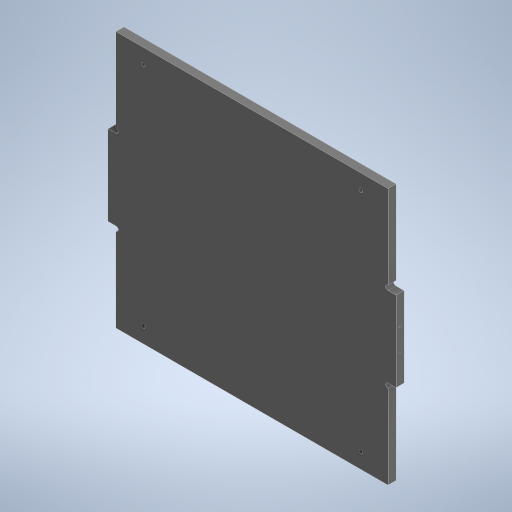
# Autodesk Inventor part: TorsoCoverFrameBasis
Saved by Autodesk Inventor 2024.2 (Build 282272000, 272)
## iProperties
Created: 2024-01-05
Part Number: TorsoCoverFrameBasis
Material: Acetal Resin, Black
Document SubType Name: Modeling
Designer: Masato Kubotera
Density: 1.425 g/cm^3
Appearance: Gray
Vendor: meviy
Mass: 132.259 g
Surface Area: 403.156 cm^2
Volume: 92.813 cm^3
Author: Masato Kubotera
Autodesk Inventor part; units mm, degrees
ref_plane "YZ Plane" through (0, 0, 0) normal (1, 0, 0) x (0, 1, 0)
ref_plane "XZ Plane" through (0, 0, 0) normal (0, 1, 0) x (-1, 0, 0)
ref_plane "XY Plane" through (0, 0, 0) normal (0, 0, 1) x (1, 0, 0)
sketch "Sketch1" plane through (0, 0, 0) normal (1, 0, 0) x (0, 1, 0)
  line L0 (-90, 80.25) -> (90, 80.25)
  line L1 (90, 80.25) -> (90, -80.25)
  line L2 (90, -80.25) -> (-90, -80.25)
  line L3 (-90, -80.25) -> (-90, 80.25)
  line L4 (-90, 80.25) -> (90, -80.25) construction
  line L5 (90, 80.25) -> (-90, -80.25) construction
  line L6 (85, 80.25) -> (85, 25)
  line L7 (85, 25) -> (90, 25)
  line L8 (0, 80.25) -> (0, -80.25)
  line L9 (90, 0) -> (-90, 0) construction
  arc A0 (85, 28) -> (85, 25) centre (85, 26.5) ccw
  line L10 (85, -80.25) -> (85, -25)
  line L11 (85, -25) -> (90, -25)
  arc A1 (85, -25) -> (85, -28) centre (85, -26.5) ccw
  line L12 (-90, 80.25) -> (-90, -80.25)
  line L13 (-85, 80.25) -> (-85, 25)
  line L14 (-85, 25) -> (-90, 25)
  arc A2 (-85, 25) -> (-85, 28) centre (-85, 26.5) ccw
  line L15 (-85, -80.25) -> (-85, -25)
  line L16 (-85, -25) -> (-90, -25)
  arc A3 (-85, -28) -> (-85, -25) centre (-85, -26.5) ccw
  circle A4 centre (68, 70.75) radius 3 construction
  arc A5 (68, 72.85) -> (68, 68.65) centre (68, 70.75) ccw construction
  line L17 (68, 72.85) -> (71.5201, 72.85) construction
  arc A6 (71.5201, 68.65) -> (71.5201, 72.85) centre (75.5, 70.75) ccw construction
  line L18 (68, 70.75) -> (75.5, 70.75) construction
  line L19 (68, 68.65) -> (71.5201, 68.65) construction
  circle A7 centre (68, -70.75) radius 3 construction
  arc A8 (68, -68.65) -> (68, -72.85) centre (68, -70.75) ccw construction
  line L20 (68, -72.85) -> (71.5201, -72.85) construction
  arc A9 (71.5201, -72.85) -> (71.5201, -68.65) centre (75.5, -70.75) ccw construction
  line L21 (68, -70.75) -> (75.5, -70.75) construction
  line L22 (68, -68.65) -> (71.5201, -68.65) construction
  circle A10 centre (-68, 70.75) radius 3 construction
  arc A11 (-68, 68.65) -> (-68, 72.85) centre (-68, 70.75) ccw construction
  line L23 (-68, 72.85) -> (-71.5201, 72.85) construction
  arc A12 (-71.5201, 72.85) -> (-71.5201, 68.65) centre (-75.5, 70.75) ccw construction
  line L24 (-68, 70.75) -> (-75.5, 70.75) construction
  line L25 (-68, 68.65) -> (-71.5201, 68.65) construction
  arc A13 (-68, -72.85) -> (-68, -68.65) centre (-68, -70.75) ccw construction
  circle A14 centre (-68, -70.75) radius 3 construction
  line L26 (-68, -72.85) -> (-71.5201, -72.85) construction
  line L27 (-68, -70.75) -> (-75.5, -70.75) construction
  arc A15 (-71.5201, -68.65) -> (-71.5201, -72.85) centre (-75.5, -70.75) ccw construction
  line L28 (-68, -68.65) -> (-71.5201, -68.65) construction
  line L29 (90, 7) -> (85, 7) construction
  line L30 (90, -7) -> (85, -7) construction
  line L31 (28.3579, -70.25) -> (-28.3579, -70.25)
  line L32 (31.8934, -71.7145) -> (40.4289, -80.25)
  line L33 (-31.8934, -71.7145) -> (-40.4289, -80.25)
  arc A16 (38.9645, -78.7855) -> (42.5, -80.25) centre (42.5, -75.25) ccw
  arc A17 (31.8934, -71.7145) -> (28.3579, -70.25) centre (28.3579, -75.25) ccw
  arc A18 (-28.3579, -70.25) -> (-31.8934, -71.7145) centre (-28.3579, -75.25) ccw
  arc A19 (-42.5, -80.25) -> (-38.9645, -78.7855) centre (-42.5, -75.25) ccw
  point P0 (0, 0)
  point P1 (-85, -80.25)
  point P2 (85, -80.25)
  point P3 (-85, 80.25)
  point P4 (30.4289, -70.25)
  point P5 (-30.4289, -70.25)
  point P6 (0, -70.25)
  point P7 (-40.4289, -80.25)
  point P8 (-42.5, -80.25)
  point P9 (-38.9645, -78.7855)
  dimension "d0" = 180
  dimension "d1" = 160.5
  dimension "d2" = 1.5
  dimension "d3" = 5
  dimension "d4" = 50
  dimension "d15" = 6
  dimension "d16" = 4.2
  dimension "d17" = 9
  dimension "d18" = 5
  dimension "d19" = 5
  dimension "d27" = 5
  dimension "d28" = 14
  dimension "d30" = 135
  dimension "d31" = 10
  dimension "d34" = 5
  dimension "d35" = 5
  dimension "d36" = 85
  constraints: 68 end point, 46 symmetric about line, 32 point on circle, 20 centre point, 19 point on line, 9 tangent, 8 coincident, 6 horizontal, 6 midpoint, 2 parallel, 1 equal radius, 1 perpendicular, 1 vertical, 14 other
  measures "d0" distance of L1.end L2.end
  measures "d1" distance of L0.end L1.end
  measures "d2" radius of A0
  measures "d3" distance between parallel lines of L1 L6
  measures "d4" distance between parallel lines of L11 L7
  measures "d15" diameter of A4
  measures "d16" diameter of A5
  measures "d17" diameter of A6
  measures "d18" distance edge to line of A6 L0
  measures "d19" distance edge to line of A6 L6
  measures "d27" distance of L29.start L29.end
  measures "d28" distance of L30.start L29.start
  measures "d30" angle of L31 L32
  measures "d31" distance between parallel lines of L2 L31
  measures "d34" radius of A16
  measures "d35" radius of A17
  measures "d36" distance of A16.end A19.start
extrude "Extrusion1" add sketch "Sketch1" along normal blind 5 contours L0 L6 A0 L7 L1 L11 A1 L10 L2 A16 L32 A17 L31 L8 | L31 A17 L32 L2 L8 | L32 A16 L2
sketch "Sketch2" plane through (0, 90, 25) normal (0, 1, 0) x (1, 0, 0)
  line L0 (5, 32) -> (0, 32) construction
  line L1 (5, 18) -> (0, 18) construction
  line L2 (0, 25) -> (5, 25) construction
  line L3 (5, 50) -> (5, 0) projected
  line L4 (0, 50) -> (0, 0) projected
  point P0 (2.5, 32)
  point P1 (2.5, 18)
  constraints: 6 end point, 2 midpoint, 2 point on line, 1 horizontal, 2 other
hole "Hole1" at (2.5, 90, -7) at (2.5, 90, 7) direction (0, -1, 0) diameter 1.567 depth 5 thread size "M2x0.4" class "6H" standard "ANSI Metric M Profile"
hole "Hole2" at (0, 68, 70.75) at (0, 68, -70.75) at (0, -68, -70.75) at (0, -68, 70.75) direction (1, 0, 0) diameter 2.459 end through all thread size "M3x0.5" class "6H" standard "ANSI Metric M Profile"
mirror "Mirror1" about plane through (0, 0, 0) normal (0, 1, 0)
equation "\"d19\" = d18"
equation "\"d35\" = d34"
equation "\"d13\" = d27"
body "Solid1"
